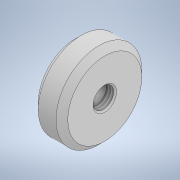
# Autodesk Inventor part: 711131
Saved by Autodesk Inventor 2022 (Build 260153000, 153)
## iProperties
Created: 2021-10-22
Part Number: 711131
Material: Типовые
Document SubType Name: Modeling
Designer: RaNSiD
Density: 1 g/cm^3
Appearance: По умолчанию
Mass: 22.5337 g
Surface Area: 51.5454 cm^2
Volume: 22.5337 cm^3
Author: RaNSiD
Autodesk Inventor part; units mm, degrees
ref_plane "YZ Plane" through (0, 0, 0) normal (1, 0, 0) x (0, 1, 0)
ref_plane "XZ Plane" through (0, 0, 0) normal (0, 1, 0) x (-1, 0, 0)
ref_plane "XY Plane" through (0, 0, 0) normal (0, 0, 1) x (1, 0, 0)
sketch "Эскиз3" plane through (0, 0, 0) normal (0, 0, 1) x (1, 0, 0)
  line L0 (0, 0) -> (20, 0)
  line L1 (20, 0) -> (20, 25)
  line L2 (16, 29) -> (4, 29)
  line L3 (0, 25) -> (0, 0)
  line L4 (4, 29) -> (0, 25)
  line L5 (16, 29) -> (20, 25)
  point P0 (20, 29)
  point P1 (0, 29)
  dimension "d18" = 20
  dimension "d19" = 29
  dimension "d20" = 4
  dimension "d21" = 4
  dimension "d22" = 4
  dimension "d23" = 4
  constraints: 12 end point, 4 point on line, 2 parallel, 1 horizontal, 1 perpendicular
  measures "d18" distance of point (0, 29) point (20, 29)
  measures "d19" distance of point (20, 29) L0.end
  measures "d20" distance of L2.end point (0, 29)
  measures "d21" distance of L3.start point (0, 29)
  measures "d22" distance of L2.start point (20, 29)
  measures "d23" distance of L1.end point (20, 29)
revolve "Вращение2" add sketch "Эскиз3" angle 360 about axis through (0, 0, 0) along (1, 0, 0)
sketch "Эскиз4" plane through (20, 0, 0) normal (1, 0, 0) x (0, 0, -1)
  point P0 (0, 0)
  point P1 (0, 0)
  constraints: 1 coincident
hole "Отверстие2" at (20, 0, 0) direction (-1, 0, 0) diameter 14 depth 6 tip angle 150 countersink diameter 16 countersink angle 90
thread "Резьба3" size "M14x2" class "6H" standard "ANSI Metric M Profile" full length
equation "\"d21\" = d20"
equation "\"d22\" = d20"
equation "\"d23\" = d22"
